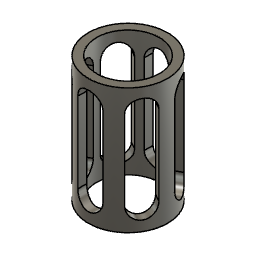
GasChargingCryoarmGuide v5 (Autodesk Fusion 360 design; units mm, degrees)
Autodesk Fusion 360 part; units mm, degrees
note: some values were not read from the file. Set by a fixed rule: which sketch regions a step uses.
sketch "Skizze1" plane through (0, 0, 0) normal (0, 1, 0) x (1, 0, 0)
  circle A0 centre (0, 0) radius 7.9
  circle A1 centre (0, 0) radius 6.25
  dimension "d1" = 15.8
  dimension "d2" = 12.5
  constraint coincident A0.centre A1.centre
  measures "d1" diameter of A0
  measures "d2" diameter of A1
extrude "Extrusion1" add sketch "Skizze1" along normal blind 25 makes body 1
ref_plane "Arbeitsebene1" through (0, 24.007, 7.9) normal (0, 0, 1) x (-1, 0, 0)
sketch "Skizze2" plane through (0, 24.3109, 7.9) normal (0, 0, 1) x (1, 0, 0)
  line L0 (0, 0.6891) -> (0, -24.3109) construction
  line L1 (7.9, 0.6891) -> (-7.9, 0.6891)
  line L2 (7.9, -24.3109) -> (-7.9, -24.3109)
  circle A0 centre (0, -3.8109) radius 2.5
  circle A1 centre (0, -11.8109) radius 2.5
  circle A2 centre (0, -19.8109) radius 2.5
  line L3 (0, -20.1067) -> (0, -3.8109)
  line L4 (2.5, -3.8109) -> (-2.5, -3.8109)
  line L5 (-2.5, -3.8109) -> (-2.5, -19.8109)
  line L6 (-2.5, -19.8109) -> (2.5, -19.8109)
  line L7 (2.5, -19.8109) -> (2.5, -3.8109)
  line L8 (2.5, -3.8109) -> (-2.5, -19.8109) construction
  line L9 (-2.5, -3.8109) -> (2.5, -19.8109) construction
  point P0 (0, -11.8109)
  dimension "d22" = 5
  dimension "d25" = 0
  dimension "d26" = -16
  dimension "d27" = 4.5
  dimension "d28" = 5
  constraint vertical L0
  constraint midpoint L0.start L1
  constraint midpoint L0.end L2
  constraint coincident L0 A0.centre
  constraint vertical L3
  constraint coincident A0.centre L3.end
  constraint horizontal L4
  constraint perpendicular L4 L5
  constraint parallel L4 L6
  constraint parallel L5 L7
  constraint coincident L8 P0
  constraint coincident L9 P0
  constraint coincident A0 L4.start
  constraint coincident P0 A1.centre
  measures "d22" diameter of A0
  measures "d27" distance of L1 A0.centre
  measures "d28" distance of L5.end L6.end
extrude "Extrusion2" cut sketch "Skizze2" against normal through all bodies 1
pattern_circular "C-Anordnung1" count 6 over 360 about axis through (0, 1.75, 0) along (0, 1, 0) of "Extrusion2"
copy_body "Körper->Berechn1" bodies 1 removing the originals makes body 2 in component "Component"
component "Component" placed x (1, 0, 0) y (0, 1, 0) z (0, 0, 1) at (0, 0, 0)
